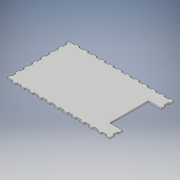
# Autodesk Inventor part: cara_superior
Saved by Autodesk Inventor 2019 (Build 230136000, 136)
## iProperties
Created: 2018-06-06
Part Number: cara_superior
Material: Generic
Document SubType Name: Modeling
Designer: seba
Density: 1 g/cm^3
Appearance: Default
Author: seba
Autodesk Inventor part; units mm, degrees
ref_plane "YZ Plane" through (0, 0, 0) normal (1, 0, 0) x (0, 1, 0)
ref_plane "XZ Plane" through (0, 0, 0) normal (0, 1, 0) x (-1, 0, 0)
ref_plane "XY Plane" through (0, 0, 0) normal (0, 0, 1) x (1, 0, 0)
sketch "Sketch1" plane through (0, 0, 0) normal (0, 1, 0) x (-1, 0, 0)
  point P0 (0, 0)
sketch "Sketch2" plane through (0, 0, 0) normal (0, 1, 0) x (-1, 0, 0)
  line L0 (0, 0) -> (3, 0)
  line L1 (3, 0) -> (3, -10)
  line L2 (3, -10) -> (0, -10)
  line L3 (0, -10) -> (0, -20)
  line L4 (0, -20) -> (3, -20)
  line L5 (3, -20) -> (3, -30)
  line L6 (3, -30) -> (0, -30)
  line L7 (0, -30) -> (0, -40)
  line L8 (0, -40) -> (3, -40)
  line L9 (3, -40) -> (3, -50)
  line L10 (3, -50) -> (0, -50)
  line L11 (0, -50) -> (0, -60)
  line L12 (0, -60) -> (3, -60)
  line L13 (3, -60) -> (3, -70)
  line L14 (3, -70) -> (0, -70)
  line L15 (0, -70) -> (0, -80)
  line L16 (0, -80) -> (3, -80)
  line L17 (3, -80) -> (3, -90)
  line L18 (3, -90) -> (0, -90)
  line L19 (0, -90) -> (0, -100)
  line L20 (0, -100) -> (3, -100)
  line L21 (3, -100) -> (3, -107)
  line L22 (3, -107) -> (0, -107)
  line L23 (0, -107) -> (-10, -107)
  line L24 (-10, -107) -> (-10, -110)
  line L25 (-10, -110) -> (-20, -110)
  line L26 (-20, -110) -> (-20, -107)
  line L27 (-20, -107) -> (-30, -107)
  line L28 (-30, -107) -> (-30, -110)
  line L29 (-30, -110) -> (-40, -110)
  line L30 (-40, -110) -> (-40, -107)
  line L31 (-40, -107) -> (-50, -107)
  line L32 (-50, -107) -> (-50, -110)
  line L33 (-50, -110) -> (-60, -110)
  line L34 (-60, -110) -> (-60, -107)
  line L35 (-60, -107) -> (-70, -107)
  line L36 (-70, -107) -> (-70, -110)
  line L37 (-70, -110) -> (-80, -110)
  line L38 (-80, -110) -> (-80, -107)
  line L39 (-80, -107) -> (-90, -107)
  line L40 (-90, -107) -> (-90, -110)
  line L41 (-90, -110) -> (-100, -110)
  line L42 (-100, -110) -> (-100, -107)
  line L43 (-100, -107) -> (-110, -107)
  line L44 (-110, -107) -> (-110, -110)
  line L45 (-110, -110) -> (-120, -110)
  line L46 (-120, -110) -> (-120, -107)
  line L47 (-120, -107) -> (-130, -107)
  line L48 (-130, -107) -> (-130, -110)
  line L49 (-130, -110) -> (-140, -110)
  line L50 (-140, -110) -> (-140, -107)
  line L51 (-140, -107) -> (-150, -107)
  line L52 (-150, -107) -> (-150, -110)
  line L53 (-150, -110) -> (-160, -110)
  line L54 (-160, -110) -> (-160, -107)
  line L55 (-160, -107) -> (-170, -107)
  line L56 (-170, -107) -> (-170, -110)
  line L57 (-170, -110) -> (-180, -110)
  line L58 (-180, -110) -> (-180, -107)
  line L59 (-180, -107) -> (-190, -107)
  line L60 (-190, -107) -> (-190, -110)
  line L61 (-190, -110) -> (-200, -110)
  line L62 (-200, -110) -> (-200, -107)
  line L63 (-200, -107) -> (-210, -107)
  line L64 (-210, -107) -> (-210, -110)
  line L65 (-210, -110) -> (-220, -110)
  line L66 (-220, -110) -> (-220, -107)
  line L67 (-220, -107) -> (-230, -107)
  line L68 (-230, -107) -> (-230, -110)
  line L69 (-230, -110) -> (-240, -110)
  line L70 (-240, -110) -> (-240, -100)
  line L71 (-240, -100) -> (-237, -100)
  line L72 (-237, -100) -> (-237, -90)
  line L73 (-237, -90) -> (-240, -90)
  line L74 (-240, -90) -> (-240, -80)
  line L75 (-240, -80) -> (-210, -80)
  line L76 (-210, -80) -> (-210, 10)
  line L77 (-210, 10) -> (-240, 10)
  line L78 (-240, 10) -> (-240, 20)
  line L79 (-240, 20) -> (-237, 20)
  line L80 (-237, 20) -> (-237, 30)
  line L81 (-237, 30) -> (-240, 30)
  line L82 (-240, 30) -> (-240, 40)
  line L83 (-240, 40) -> (-230, 40)
  line L84 (-230, 40) -> (-230, 37)
  line L85 (-230, 37) -> (-220, 37)
  line L86 (-220, 37) -> (-220, 40)
  line L87 (-220, 40) -> (-210, 40)
  line L88 (-210, 40) -> (-210, 37)
  line L89 (-210, 37) -> (-200, 37)
  line L90 (-200, 37) -> (-200, 40)
  line L91 (-200, 40) -> (-190, 40)
  line L92 (-190, 40) -> (-190, 37)
  line L93 (-190, 37) -> (-180, 37)
  line L94 (-180, 37) -> (-180, 40)
  line L95 (-180, 40) -> (-170, 40)
  line L96 (-170, 40) -> (-170, 37)
  line L97 (-170, 37) -> (-160, 37)
  line L98 (-160, 37) -> (-160, 40)
  line L99 (-160, 40) -> (-150, 40)
  line L100 (-150, 40) -> (-150, 37)
  line L101 (-150, 37) -> (-140, 37)
  line L102 (-140, 37) -> (-140, 40)
  line L103 (-140, 40) -> (-130, 40)
  line L104 (-130, 40) -> (-130, 37)
  line L105 (-130, 37) -> (-120, 37)
  line L106 (-120, 37) -> (-120, 40)
  line L107 (-120, 40) -> (-110, 40)
  line L108 (-110, 40) -> (-110, 37)
  line L109 (-110, 37) -> (-100, 37)
  line L110 (-100, 37) -> (-100, 40)
  line L111 (-100, 40) -> (-90, 40)
  line L112 (-90, 40) -> (-90, 37)
  line L113 (-90, 37) -> (-80, 37)
  line L114 (-80, 37) -> (-80, 40)
  line L115 (-80, 40) -> (-70, 40)
  line L116 (-70, 40) -> (-70, 37)
  line L117 (-70, 37) -> (-60, 37)
  line L118 (-60, 37) -> (-60, 40)
  line L119 (-60, 40) -> (-50, 40)
  line L120 (-50, 40) -> (-50, 37)
  line L121 (-50, 37) -> (-40, 37)
  line L122 (-40, 37) -> (-40, 40)
  line L123 (-40, 40) -> (-30, 40)
  line L124 (-30, 40) -> (-30, 37)
  line L125 (-30, 37) -> (-20, 37)
  line L126 (-20, 37) -> (-20, 40)
  line L127 (-20, 40) -> (-10, 40)
  line L128 (-10, 40) -> (-10, 37)
  line L129 (-10, 37) -> (3, 37)
  line L130 (3, 37) -> (3, 30)
  line L131 (3, 30) -> (0, 30)
  line L132 (0, 30) -> (0, 20)
  line L133 (3, 10) -> (0, 10)
  line L134 (0, 10) -> (0, 0)
  line L135 (3, 20) -> (3, 10)
  line L136 (0, 20) -> (3, 20)
  dimension "d1" = 10
  dimension "d3" = 10
  dimension "d4" = 10
  dimension "d5" = 10
  dimension "d6" = 10
  dimension "d7" = 10
  dimension "d8" = 10
  dimension "d9" = 10
  dimension "d10" = 10
  dimension "d11" = 10
  dimension "d12" = 7
  dimension "d42" = 3
  dimension "d43" = 10
  dimension "d44" = 10
  dimension "d45" = 10
  dimension "d46" = 10
  dimension "d47" = 10
  dimension "d48" = 10
  dimension "d49" = 10
  dimension "d50" = 10
  dimension "d51" = 10
  dimension "d52" = 10
  dimension "d53" = 10
  dimension "d54" = 10
  dimension "d55" = 10
  dimension "d56" = 10
  dimension "d57" = 10
  dimension "d58" = 10
  dimension "d59" = 10
  dimension "d60" = 10
  dimension "d61" = 10
  dimension "d62" = 10
  dimension "d63" = 10
  dimension "d64" = 10
  dimension "d66" = 10
  dimension "d67" = 10
  dimension "d68" = 10
  dimension "d69" = 3
  dimension "d70" = 10
  dimension "d71" = 10
  dimension "d73" = 10
  dimension "d74" = 10
  dimension "d75" = 10
  dimension "d79" = 10
  dimension "d80" = 10
  dimension "d81" = 10
  dimension "d82" = 10
  dimension "d83" = 10
  dimension "d84" = 10
  dimension "d85" = 10
  dimension "d86" = 10
  dimension "d87" = 10
  dimension "d88" = 10
  dimension "d89" = 10
  dimension "d90" = 10
  dimension "d91" = 10
  dimension "d92" = 10
  dimension "d93" = 10
  dimension "d94" = 10
  dimension "d95" = 10
  dimension "d96" = 10
  dimension "d97" = 10
  dimension "d98" = 10
  dimension "d99" = 10
  constraints: 274 end point, 93 point on line, 73 perpendicular, 14 horizontal, 5 vertical
  measures "d1" distance of L0.end L1.end
  measures "d3" distance of L4.end L5.end
  measures "d4" distance of L2.end L3.end
  measures "d5" distance of L6.end L7.end
  measures "d6" distance of L8.end L9.end
  measures "d7" distance of L10.end L11.end
  measures "d8" distance of L12.end L13.end
  measures "d9" distance of L14.end L15.end
  measures "d10" distance of L16.end L17.end
  measures "d11" distance of L18.end L19.end
  measures "d12" distance of L20.end L21.end
  measures "d42" distance of L23.end L24.end
  measures "d43" distance of L22.end L23.end
  measures "d44" distance of L24.end L25.end
  measures "d45" distance of L26.end L27.end
  measures "d46" distance of L28.end L29.end
  measures "d47" distance of L30.end L31.end
  measures "d48" distance of L32.end L33.end
  measures "d49" distance of L34.end L35.end
  measures "d50" distance of L36.end L37.end
  measures "d51" distance of L38.end L39.end
  measures "d52" distance of L40.end L41.end
  measures "d53" distance of L42.end L43.end
  measures "d54" distance of L44.end L45.end
  measures "d55" distance of L46.end L47.end
  measures "d56" distance of L48.end L49.end
  measures "d57" distance of L50.end L51.end
  measures "d58" distance of L52.end L53.end
  measures "d59" distance of L54.end L55.end
  measures "d60" distance of L56.end L57.end
  measures "d61" distance of L58.end L59.end
  measures "d62" distance of L60.end L61.end
  measures "d63" distance of L62.end L63.end
  measures "d64" distance of L64.end L65.end
  measures "d66" distance of L66.end L67.end
  measures "d67" distance of L68.end L69.end
  measures "d68" distance of L69.end L70.end
  measures "d69" distance of L70.end L71.end
  measures "d70" distance of L71.end L72.end
  measures "d71" distance of L73.end L74.end
  measures "d73" distance of L77.end L78.end
  measures "d74" distance of L79.end L80.end
  measures "d75" distance of L81.end L82.end
  measures "d79" distance of L82.end L83.end
  measures "d80" distance of L84.end L85.end
  measures "d81" distance of L86.end L87.end
  measures "d82" distance of L88.end L89.end
  measures "d83" distance of L90.end L91.end
  measures "d84" distance of L92.end L93.end
  measures "d85" distance of L94.end L95.end
  measures "d86" distance of L96.end L97.end
  measures "d87" distance of L98.end L99.end
  measures "d88" distance of L100.end L101.end
  measures "d89" distance of L102.end L103.end
  measures "d90" distance of L104.end L105.end
  measures "d91" distance of L106.end L107.end
  measures "d92" distance of L108.end L109.end
  measures "d93" distance of L110.end L111.end
  measures "d94" distance of L112.end L113.end
  measures "d95" distance of L114.end L115.end
  measures "d96" distance of L116.end L117.end
  measures "d97" distance of L118.end L119.end
  measures "d98" distance of L120.end L121.end
  measures "d99" distance of L122.end L123.end
sketch "Sketch3" plane through (0, 0, 0) normal (0, 1, 0) x (-1, 0, 0)
  point P0 (0, 0)
extrude "Extrusion1" add sketch "Sketch2" along normal blind 3
body "Solid1"
